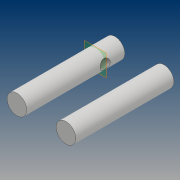
# Autodesk Inventor part: 槌子支架
Saved by Autodesk Inventor 2018 (Build 220112000, 112)
## iProperties
Created: 2020-11-30
Part Number: 槌子支架
Material: 一般
Document SubType Name: Modeling
Designer: 88697
Density: 1 g/cm^3
Appearance: 預設
Author: 88697
Autodesk Inventor part; units mm, degrees
ref_plane "YZ Plane" through (0, 0, 0) normal (1, 0, 0) x (0, 1, 0)
ref_plane "XZ Plane" through (0, 0, 0) normal (0, 1, 0) x (-1, 0, 0)
ref_plane "XY Plane" through (0, 0, 0) normal (0, 0, 1) x (1, 0, 0)
sketch "草圖1" plane through (0, 0, 0) normal (0, 1, 0) x (-1, 0, 0)
  line L0 (0, 0) -> (-15, 0) construction
  line L1 (-15, 0) -> (-15, -10) construction
  line L2 (-15, -10) -> (0, -10) construction
  line L3 (0, -10) -> (0, 0) construction
  line L4 (-25, 0) -> (-40, 0) construction
  line L5 (-40, 0) -> (-40, -10) construction
  line L6 (-40, -10) -> (-25, -10) construction
  line L7 (-25, -10) -> (-25, 0) construction
  circle A0 centre (-7.5, -5) radius 5
  circle A1 centre (-32.5, -5) radius 5
  dimension "d0" = 15
  dimension "d1" = 15
  dimension "d2" = 10
  dimension "d3" = 10
  dimension "d4" = 10
  dimension "d5" = 10
  dimension "d6" = 7.5
  dimension "d7" = 25
  dimension "d8" = 5
  dimension "d9" = 5
  constraints: 16 end point, 4 parallel, 2 centre point, 2 horizontal, 2 perpendicular, 2 point on line
  measures "d0" distance of L0.start L0.end
  measures "d1" distance of L4.start L4.end
  measures "d2" distance between parallel lines of L1 L7
  measures "d3" distance between parallel lines of L0 L2
  measures "d4" diameter of A0
  measures "d5" diameter of A1
  measures "d6" distance from line of L3 A0.centre
  measures "d7" distance of A1.centre A0.centre
  measures "d8" distance from line of L2 A0.centre
  measures "d9" distance from line of A1.centre L6
extrude "擠出1" add sketch "草圖1" along normal blind 50
ref_plane "工作平面1" through (7.5, 40, -5) normal (0, 1, 0) x (1, 0, 0)
sketch "草圖4" plane through (7.5, 40, -5) normal (0, 1, 0) x (1, 0, 0)
  line L0 (0, 0) -> (25, 0)
  line L1 (25, 0) -> (25, 2.5)
  line L2 (25, 2.5) -> (0, 2.5)
  line L3 (0, 2.5) -> (0, 0)
  circle A0 centre (25, 0) radius 5 projected
  circle A1 centre (0, 0) radius 5 projected
  point P0 (-7.5, -5)
  dimension "d17" = 0
  dimension "d18" = 0
  dimension "d19" = 2.5
  dimension "d20" = 0
  constraints: 8 end point, 2 parallel, 1 horizontal, 1 perpendicular
  measures "d17" distance from line of A0.centre L1
  measures "d18" distance from line of A1.centre L3
  measures "d19" distance of L2.end L0.start
  measures "d20" distance from line of L0 A1.centre
revolve "迴轉2" cut sketch "草圖4" angle 360 about axis through (7.5, 40, -5) along (1, 0, 0) picked at (1.4434, 1.6667) picked at (23.5566, 1.6667) contours L3 L2 A1 L0 | A1 L2 A0 L0 | A0 L2 L1 L0
